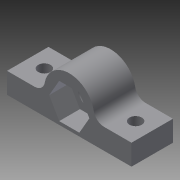
# Autodesk Inventor part: motor_bracket
Saved by Autodesk Inventor 2015 (Build 190159000, 159)
## iProperties
Created: 2015-12-01
Part Number: motor_bracket
Material: Generic
Document SubType Name: Modeling
Designer: jufranz
Density: 1 g/cm^3
Appearance: Default
Author: jufranz
Autodesk Inventor part; units mm, degrees
ref_plane "YZ Plane" through (0, 0, 0) normal (1, 0, 0) x (0, 1, 0)
ref_plane "XZ Plane" through (0, 0, 0) normal (0, 1, 0) x (-1, 0, 0)
ref_plane "XY Plane" through (0, 0, 0) normal (0, 0, 1) x (1, 0, 0)
sketch "Sketch1" plane through (0, 0, 0) normal (0, 1, 0) x (-1, 0, 0)
  line L0 (15, 5) -> (-15, 5)
  line L1 (-15, 5) -> (-15, -5)
  line L2 (-15, -5) -> (15, -5)
  line L3 (15, -5) -> (15, 5)
  point P0 (0, 0)
  point P1 (15, 0)
  point P2 (0, 5)
  dimension "d0" = 30
  dimension "d1" = 10
  constraints: 8 end point, 2 midpoint, 2 parallel, 1 horizontal, 1 horizontal alignment, 1 perpendicular, 1 vertical alignment
  measures "d0" distance of L0.start L0.end
  measures "d1" distance between parallel lines of L2 L0
extrude "Extrusion1" add sketch "Sketch1" along normal blind 5
sketch "Sketch3" plane through (0, 5, 0) normal (0, 1, 0) x (1, 0, 0)
  line L0 (-15, -5) -> (15, -5) projected
  line L1 (-6, 5) -> (6, 5)
  line L2 (6, 5) -> (6, -5)
  line L3 (6, -5) -> (-6, -5)
  line L4 (-6, -5) -> (-6, 5)
  line L5 (15, 5) -> (-15, 5) projected
  point P0 (0, 0)
  point P1 (0, 5)
  dimension "d13" = 12
  dimension "d14" = 6
  constraints: 8 end point, 2 midpoint, 2 parallel, 1 horizontal, 1 perpendicular, 1 point on line
  measures "d13" distance between parallel lines of L4 L2
  measures "d14" distance from line of L4 point (0, 0)
extrude "Extrusion2" add sketch "Sketch3" along normal blind 7
sketch "Sketch4" plane through (-15, 0, 5) normal (0, 0, 1) x (1, 0, 0)
  line L0 (9, 12) -> (21, 12) projected
  line L1 (9, 5) -> (9, 12) projected
  line L2 (0, 5) -> (9, 5) projected
  line L3 (0, 0) -> (30, 0) projected
  point P0 (15, 0)
  point P1 (15, 5)
  dimension "d18" = 6
  dimension "d45" = 5
  measures "d18" distance from line of L1 point (15, 5)
  measures "d45" distance from line of L3 point (15, 5)
hole "Hole2" at (0, 5, 5) direction (0, 0, -1) diameter 6 end through all
sketch "Sketch5" plane through (-15, 0, 5) normal (0, 0, 1) x (1, 0, 0)
  line L0 (9, 12) -> (21, 12) projected
  line L1 (21, 5) -> (21, 12) projected
  line L2 (0, 5) -> (9, 5) projected
  line L3 (0, 0) -> (30, 0) projected
  line L4 (19.8497, 5) -> (17.4249, 0.8)
  line L5 (17.4249, 0.8) -> (12.5751, 0.8)
  line L6 (12.5751, 0.8) -> (10.1503, 5)
  line L7 (10.1503, 5) -> (12.5751, 9.2)
  line L8 (12.5751, 9.2) -> (17.4249, 9.2)
  line L9 (17.4249, 9.2) -> (19.8497, 5)
  point P0 (15, 0)
  point P1 (15, 5)
  point P2 (13.175, 20)
  point P3 (16.825, 20)
  point P4 (20, 13.175)
  point P5 (20, 16.825)
  point P6 (15, 5)
  dimension "d46" = 5
  dimension "d47" = 8.4
  dimension "d48" = 6
  constraints: 12 end point, 1 coincident, 15 other
  measures "d46" distance from line of L3 point (15, 5)
  measures "d47" distance between parallel lines of L9 L6
extrude "Extrusion3" cut sketch "Sketch5" against normal blind 5
fillet "Fillet2" radius 6 2 edges at (-6, 12, 0) (6, 12, 0)
fillet "Fillet3" radius 2.5 2 edges at (6, 5, 0) (-6, 5, 0)
sketch "Sketch6" plane through (0, 0, 0) normal (0, -1, 0) x (1, 0, 0)
  line L0 (-15, -5) -> (-15, 5) projected
  line L1 (15, 5) -> (15, -5) projected
  point P0 (0, 0)
  point P1 (-11, 0)
  point P2 (11, 0)
  dimension "d33" = 4
  dimension "d34" = 4
  constraints: 2 horizontal alignment
  measures "d33" distance from line of L0 point (-11, 0)
  measures "d34" distance from line of L1 point (11, 0)
hole "Hole3" at (-11, 0, 0) at (11, 0, 0) direction (0, 1, 0) diameter 3 end through all
equation "\"d14\" = 0.5 * d13"
equation "\"d18\" = d17"
equation "\"d46\" = d45"
equation "\"d48\" = 0.5 * d13"
equation "\"d34\" = d33"
equation "\"d17\" = 6"
body "Solid1"
